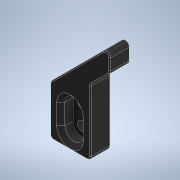
# Autodesk Inventor part: UpperAcrylicSheetHolder
Saved by Autodesk Inventor 2021 (Build 250183000, 183)
## iProperties
Created: 2020-07-17
Part Number: UpperAcrylicSheetHolder
Material: Generic
Document SubType Name: Modeling
Designer: CASE-SMALL2
Density: 1 g/cm^3
Appearance: Default
Author: CASE-SMALL2
## iProperties of the stored document _3DPrint.ipt
Created: 2020-07-17
Part Number: _3DPrint
Material: Generic
Document SubType Name: Modeling
Designer: CASE-SMALL2
Density: 1 g/cm^3
Appearance: Default
Author: CASE-SMALL2
Autodesk Inventor part; units mm, degrees
ref_plane "YZ Plane" through (0, 0, 0) normal (1, 0, 0) x (0, 1, 0)
ref_plane "XZ Plane" through (0, 0, 0) normal (0, 1, 0) x (-1, 0, 0)
ref_plane "XY Plane" through (0, 0, 0) normal (0, 0, 1) x (1, 0, 0)
sketch "Sketch1" plane through (0, 0, 0) normal (0, 0, 1) x (1, 0, 0)
  line L0 (0, 0) -> (20, 0)
  line L1 (20, 0) -> (20, 24)
  line L2 (20, 24) -> (0, 24)
  line L3 (0, 24) -> (0, 0)
  line L4 (0, 24) -> (28.2843, 52.2843)
  line L5 (29.598, 42.2843) -> (29.598, 52.2843)
  line L6 (20, 24) -> (20, 32.6863)
  line L7 (20, 32.6863) -> (29.598, 42.2843)
  line L8 (10, 0) -> (10, 46.8926) construction
  circle A0 centre (10, 17) radius 2.4
  circle A1 centre (10, 7) radius 2.4
  line L9 (28.2843, 52.2843) -> (29.598, 52.2843)
  dimension "d0" = 24
  dimension "d1" = 20
  dimension "d3" = 8
  dimension "d4" = 45
  dimension "d6" = 4.8
  dimension "d7" = 4.8
  dimension "d8" = 7
  dimension "d9" = 7
  dimension "d10" = 10
  dimension "d12" = 40
  constraints: 20 end point, 3 parallel, 3 vertical, 2 centre point, 2 perpendicular, 2 point on line, 1 horizontal, 1 midpoint
  measures "d0" distance of L0.end L1.end
  measures "d1" distance of L1.end L2.end
  measures "d3" distance between parallel lines of L4 L7
  measures "d4" angle of L7 L2
  measures "d6" diameter of A0
  measures "d7" diameter of A1
  measures "d8" distance from line of L2 A0.centre
  measures "d9" distance from line of L0 A1.centre
  measures "d10" distance from line of L5.start L9
  measures "d12" distance of L2.end L4.end
extrude "Extrusion1" add sketch "Sketch1" along normal mid plane 10
sketch "Sketch2" plane through (0, 0, 5) normal (0, 0, 1) x (1, 0, 0)
  circle A0 centre (10, 17) radius 2.4 projected
  circle A1 centre (10, 7) radius 2.4 projected
  arc A2 (14.5, 17) -> (5.5, 17) centre (10, 17) ccw
  arc A3 (5.5, 7) -> (14.5, 7) centre (10, 7) ccw
  line L0 (5.5, 17) -> (5.5, 7)
  line L1 (14.5, 17) -> (14.5, 7)
  point P0 (0, 0)
  dimension "d15" = 9
  dimension "d16" = 9
  constraints: 4 end point, 4 point on circle, 3 tangent, 2 centre point, 1 vertical
  measures "d15" diameter of A2
  measures "d16" diameter of A3
extrude "Extrusion2" cut sketch "Sketch2" against normal blind 6
sketch "Sketch4" plane through (0, 24, -5) normal (-0.7071, 0.7071, 0) x (-0.7071, -0.7071, 0)
  line L0 (38.7328, 5) -> (-54.2059, 5) projected
  circle A0 centre (-25, 5) radius 1.9
  line L1 (0, 0) -> (0, 10) projected
  point P0 (16.9706, 5)
  dimension "d19" = 3.8
  dimension "d20" = 25
  constraints: 1 centre point, 1 point on line
  measures "d19" diameter of A0
  measures "d20" distance from line of A0.centre L1
extrude "Extrusion3" cut sketch "Sketch4" against normal through all
sketch "Sketch5" plane through (29.598, 42.2843, 5) normal (0.7071, -0.7071, 0) x (-0.7071, -0.7071, 0)
  circle A0 centre (8.8579, 5) radius 1.9 projected
  line L0 (8.8579, 8.5796) -> (11.9579, 6.7898)
  line L1 (11.9579, 6.7898) -> (11.9579, 3.2102)
  line L2 (11.9579, 3.2102) -> (8.8579, 1.4204)
  line L3 (8.8579, 1.4204) -> (5.7579, 3.2102)
  line L4 (5.7579, 3.2102) -> (5.7579, 6.7898)
  line L5 (5.7579, 6.7898) -> (8.8579, 8.5796)
  point P0 (50.8284, 5)
  dimension "d23" = 6.2
  constraints: 12 end point, 1 coincident, 1 vertical, 13 other
  measures "d23" distance between parallel lines of L5 L2
extrude "Extrusion4" cut sketch "Sketch5" against normal blind 6
fillet "Fillet1" radius 2 7 edges at (0, 0, 0) (20, 0, 0) (0, 24, 0) (20, 32.6863, 0) (29.598, 42.2843, 0) (29.598, 52.2843, 0) (28.2843, 52.2843, 0)
chamfer "Chamfer1" distance 2 angle 45 4 edges at (5.5, 12, 5) (10, 21.5, 5) (14.5, 12, 5) (10, 2.5, 5)
chamfer "Chamfer2" distance 0.5 angle 45 22 edges at (13.3856, 37.3856, -5) (29.598, 45.9423, -5) (29.4457, 42.3473, -5) (24.799, 37.4853, -5) (20.1522, 32.6232, -5) (20, 16.9289, -5) (19.4142, 0.5858, -5) (10, 0, -5) (0.5858, 0.5858, -5) (0, 12.5858, -5) (0.1522, 23.9369, -5) (13.3856, 37.3856, 5) (0.1522, 23.9369, 5) (0, 12.5858, 5) (0.5858, 0.5858, 5) (10, 0, 5) (19.4142, 0.5858, 5) (20, 16.9289, 5) (20.1522, 32.6232, 5) (24.799, 37.4853, 5) (29.4457, 42.3473, 5) (29.598, 45.9423, 5)
equation "\"d7\" = d6"
equation "\"d9\" = d8"
equation "\"d16\" = d15"
body "Solid1"
